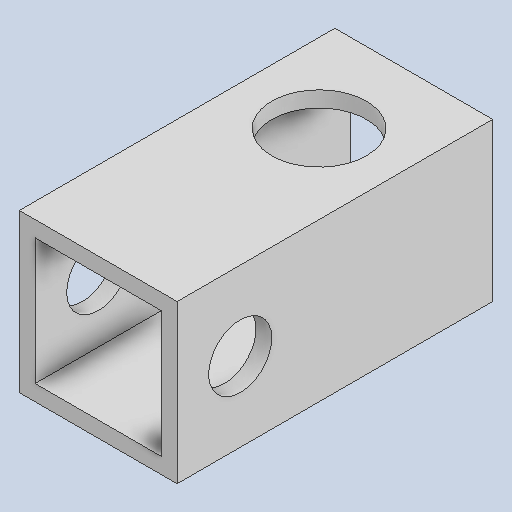
# Autodesk Inventor part: finger_k_mk_1
Saved by Autodesk Inventor 2024.1 (Build 281209000, 209)
## iProperties
Created: 2022-06-23
Part Number: finger_k_mk_1
Material: 一般
Document SubType Name: Modeling
Designer: zegi
Density: 1 g/cm^3
Appearance: 既定
Mass: 0.638319 g
Surface Area: 14.1147 cm^2
Volume: 0.638319 cm^3
Author: zegi
Autodesk Inventor part; units mm, degrees
ref_plane "YZ Plane" through (0, 0, 0) normal (1, 0, 0) x (0, 1, 0)
ref_plane "XZ Plane" through (0, 0, 0) normal (0, 1, 0) x (-1, 0, 0)
ref_plane "XY Plane" through (0, 0, 0) normal (0, 0, 1) x (1, 0, 0)
sketch "スケッチ1" plane through (0, 0, 0) normal (0, 0, 1) x (1, 0, 0)
  line L0 (0, 0) -> (10, 0)
  line L1 (10, 0) -> (10, 10)
  line L2 (10, 10) -> (0, 10)
  line L3 (0, 10) -> (0, 0)
  line L4 (1, 9) -> (9, 9)
  line L5 (9, 9) -> (9, 1)
  line L6 (9, 1) -> (1, 1)
  line L7 (1, 1) -> (1, 9)
  dimension "d0" = 10
  dimension "d1" = 10
  dimension "d2" = 1
  constraints: 16 end point, 4 parallel, 2 perpendicular, 1 horizontal, 3 other
  measures "d0" distance of L2.end L1.end
  measures "d1" distance of L1.end L0.end
  measures "d2" distance between parallel lines of L2 L4
extrude "押し出し1" add sketch "スケッチ1" along normal blind 20
sketch "スケッチ2" plane through (10, 0, 0) normal (1, 0, 0) x (0, 0, -1)
  line L0 (-20, 0) -> (-20, 10) projected
  point P0 (0, 0)
  point P1 (-16, 5)
  dimension "d5" = 4
  measures "d5" distance from line of L0 point (-16, 5)
hole "穴1" at (10, 5, 16) direction (-1, 0, 0) diameter 4 end through all
sketch "スケッチ3" plane through (0, 10, 0) normal (0, 1, 0) x (1, 0, 0)
  line L0 (10, -20) -> (0, -20) projected
  point P0 (0, 0)
  point P1 (5, -6)
  dimension "d13" = 14
  measures "d13" distance from line of L0 point (5, -6)
hole "穴2" at (5, 10, 6) direction (0, -1, 0) diameter 6 end through all
